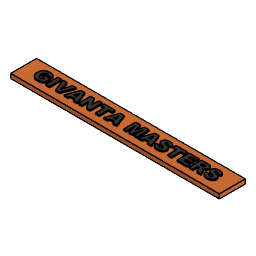
logo-strip (Autodesk Fusion 360 design; units mm, degrees)
part number: 2026-08-18-20-59-34-038
Autodesk Fusion 360 part; units mm, degrees
sketch "Sketch1" plane through (0, 0, 0) normal (0, 0, 1) x (1, 0, 0)
  line L0 (0, 0) -> (120, 0)
  dimension "d157" = 8
  text T0 "GIVANTA MASTERS" font "Arial Black" height 8 align centre spacing 1 along the path L0 letters at x, y, angle (-0.6003, 12.3001, 0) (8.7094, 12.3001, 0) (13.0587, 12.3001, 0) (21.7626, 12.3001, 0) (30.4884, 12.3001, 0) (39.7981, 12.3001, 0) (47.869, 12.3001, 0) (56.5948, 12.3001, 0) (60.322, 12.3001, 0) (70.8704, 12.3001, 0) (79.5962, 12.3001, 0) (87.6671, 12.3001, 0) (95.7381, 12.3001, 0) (103.809, 12.3001, 0) (112.5293, 12.3001, 0)
extrude "Extrude1" add sketch "Sketch1" along normal blind 0.8 text T0 makes body 1 at (97.377, 3.7963, 0) makes body 2 at (61.7881, 4.7003, 0) makes body 3 at (28.3147, 3.6835, 0) makes body 4 at (7.3379, 2.8704, 0) makes body 5 at (38.1974, 3.8581, 0) makes body 6 at (77.4225, 3.6835, 0) makes body 7 at (105.4879, 3.749, 0) makes body 8 at (91.2688, 4.0164, 0) makes body 9 at (54.4211, 3.6835, 0) makes body 10 at (15.5562, 3.4143, 0) makes body 11 at (10.452, 5.3333, 0) makes body 12 at (43.3997, 4.0164, 0) makes body 13 at (85.0771, 4.1947, 0) makes body 14 at (118.0102, 4.1947, 0)
sketch "Sketch2" plane through (0, 0, 0) normal (0, 0, 1) x (1, 0, 0)
  line L0 (-9.0873, -4.6364) -> (129.1746, -4.6364)
  line L1 (129.1746, -4.6364) -> (129.1746, 12.6364)
  line L2 (129.1746, 12.6364) -> (-9.0873, 12.6364)
  line L3 (-9.0873, 12.6364) -> (-9.0873, -4.6364)
extrude "Extrude2" add sketch "Sketch2" along normal blind 3 from surface at -3 separate body makes body 15
equation "d158 = 'GIVANTA MASTERS'"
named bodies: "Логотип (2-й цвет)", "Логотип", "Логотип (1)", "Логотип (2)", "Логотип (3)", "Логотип (4)", "Логотип (5)", "Логотип (6)", "Логотип (7)", "Логотип (8)", "Логотип (9)", "Логотип (10)", "Логотип (11)", "Логотип (12)", "Тело"
